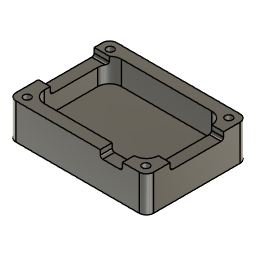
battery_holder (Autodesk Fusion 360 design; units mm, degrees)
Autodesk Fusion 360 part; units mm, degrees
sketch "Sketch1" plane through (0, 0, 0) normal (0, 0, 1) x (1, 0, 0)
  line L0 (-29, 21.25) -> (29, 21.25)
  line L1 (29, 21.25) -> (29, -21.25)
  line L2 (29, -21.25) -> (-29, -21.25)
  line L3 (-29, -21.25) -> (-29, 21.25)
  line L4 (24, -16.25) -> (-24, -16.25)
  line L5 (-24, -16.25) -> (-24, 16.25)
  line L6 (-24, 16.25) -> (24, 16.25)
  line L7 (24, 16.25) -> (24, -16.25)
  dimension "d1" = 58
  dimension "d2" = 42.5
  dimension "d3" = 21.25
  dimension "d4" = 29
  dimension "d5" = 5
  constraint horizontal L0
  constraint vertical L1
  constraint horizontal L2
  constraint vertical L3
  measures "d1" distance of L0.start L0.end
  measures "d2" distance of L0.start L2.end
  measures "d3" distance of origin L0
  measures "d4" distance of origin L3
extrude "Extrude1" add sketch "Sketch1" along normal blind 10
sketch "Sketch2" plane through (0, 0, 10) normal (0, 0, 1) x (-1, 0, 0)
  line L0 (24, -16.25) -> (-24, -16.25)
  line L1 (-24, -16.25) -> (-24, 16.25)
  line L2 (-24, 16.25) -> (24, 16.25)
  line L3 (24, 16.25) -> (24, -16.25)
  line L4 (29, 21.25) -> (-29, 21.25)
  line L5 (-29, 21.25) -> (-29, -21.25)
  line L6 (-29, -21.25) -> (29, -21.25)
  line L7 (29, -21.25) -> (29, 21.25)
  circle A0 centre (25, 17.5) radius 1.525
  line L8 (0, -2.5) -> (0, -20)
  circle A1 centre (-25, 17.5) radius 1.525
  line L9 (-20, 0) -> (-2.5, 0)
  circle A2 centre (-25, -17.5) radius 1.525
  circle A3 centre (25, -17.5) radius 1.525
  dimension "d8" = 3.05
  dimension "d9" = 4
  dimension "d10" = 3.75
  constraint symmetric A0 L8 A1
  constraint symmetric A0 L9 A3
  constraint symmetric A1 L9 A2
  measures "d8" diameter of A0
  measures "d9" distance of L7 A0.centre
  measures "d10" distance of L4 A0.centre
fillet "Fillet1" radius 5 4 edges at (-24, -16.25, 5) (-24, 16.25, 5) (24, 16.25, 5) (24, -16.25, 5)
extrude "Extrude2" cut sketch "Sketch2" against normal blind 19 contours A0 | A1 | A2 | A3
sketch "Sketch3" plane through (0, 0, 10) normal (0, 0, 1) x (-1, 0, 0)
  circle A0 centre (25, -17.5) radius 1.525
  circle A1 centre (-25, 17.5) radius 1.525
  circle A2 centre (25, 17.5) radius 1.525
  circle A3 centre (-25, -17.5) radius 1.525
  line L0 (19, -16.25) -> (-19, -16.25)
  arc A4 (-24, -11.25) -> (-19, -16.25) centre (-19, -11.25) ccw
  line L1 (-24, -11.25) -> (-24, 11.25)
  arc A5 (-19, 16.25) -> (-24, 11.25) centre (-19, 11.25) ccw
  line L2 (-19, 16.25) -> (19, 16.25)
  arc A6 (24, 11.25) -> (19, 16.25) centre (19, 11.25) ccw
  line L3 (24, 11.25) -> (24, -11.25)
  arc A7 (19, -16.25) -> (24, -11.25) centre (19, -11.25) ccw
  line L4 (29, 21.25) -> (-29, 21.25)
  line L5 (-29, 21.25) -> (-29, -21.25)
  line L6 (-29, -21.25) -> (29, -21.25)
  line L7 (29, -21.25) -> (29, 21.25)
  line L8 (24, 8.75) -> (29, 8.75)
  line L9 (29, 8.75) -> (29, -14.75)
  line L10 (29, -14.75) -> (24, -14.75)
  line L11 (24, -14.75) -> (24, 8.75)
  dimension "d15" = 6.5
  dimension "d16" = 12.5
  constraint horizontal L8
  constraint vertical L9
  constraint horizontal L10
  constraint vertical L11
  constraint coincident L7 L9.end
  constraint coincident L3 L8.start
  measures "d15" distance of L6 L10
  measures "d16" distance of L4 L8
extrude "Extrude3" cut sketch "Sketch3" against normal blind 3 contours L3 L7 L8 L9 L10 L11
sketch "Sketch4" plane through (0, 0, 10) normal (0, 0, 1) x (-1, 0, 0)
  line L0 (29, -14.75) -> (24, -14.75)
  arc A0 (19, -16.25) -> (24, -11.25) centre (19, -11.25) ccw
  line L1 (19, -16.25) -> (-19, -16.25)
  arc A1 (-24, -11.25) -> (-19, -16.25) centre (-19, -11.25) ccw
  line L2 (-24, -11.25) -> (-24, 11.25)
  arc A2 (-19, 16.25) -> (-24, 11.25) centre (-19, 11.25) ccw
  line L3 (-19, 16.25) -> (19, 16.25)
  arc A3 (24, 11.25) -> (19, 16.25) centre (19, 11.25) ccw
  line L4 (24, 11.25) -> (24, 8.75)
  line L5 (24, 8.75) -> (29, 8.75)
  line L6 (29, 8.75) -> (29, 21.25)
  line L7 (29, 21.25) -> (-29, 21.25)
  line L8 (-29, 21.25) -> (-29, -21.25)
  line L9 (-29, -21.25) -> (29, -21.25)
  line L10 (29, -21.25) -> (29, -14.75)
  circle A4 centre (-25, -17.5) radius 1.525
  circle A5 centre (25, 17.5) radius 1.525
  circle A6 centre (-25, 17.5) radius 1.525
  circle A7 centre (25, -17.5) radius 1.525
  line L11 (-24, 11.25) -> (-29, 11.25)
  line L12 (-29, 11.25) -> (-29, -11.25)
  line L13 (-29, -11.25) -> (-24, -11.25)
  line L14 (-24, -11.25) -> (-24, 11.25)
  line L15 (24, -14.75) -> (24, -11.25)
  dimension "d19" = 22.5
  constraint horizontal L11
  constraint vertical L12
  constraint horizontal L13
  constraint vertical L14
  constraint coincident L8 L12.end
  constraint coincident L2.end A2.end
  measures "d19" distance of L11.end L12.end
extrude "Extrude4" cut sketch "Sketch4" against normal blind 3 contours L2 L8 L11 L12 L13 L14
sketch "Sketch6" plane through (0, 0, 10) normal (0, 0, 1) x (-1, 0, 0)
  line L0 (-29, 11.25) -> (-24, 11.25)
  arc A0 (-19, 16.25) -> (-24, 11.25) centre (-19, 11.25) ccw
  line L1 (-19, 16.25) -> (19, 16.25)
  arc A1 (24, 11.25) -> (19, 16.25) centre (19, 11.25) ccw
  line L2 (24, 11.25) -> (24, 8.75)
  line L3 (24, 8.75) -> (29, 8.75)
  line L4 (29, 8.75) -> (29, 21.25)
  line L5 (29, 21.25) -> (-29, 21.25)
  line L6 (-29, 21.25) -> (-29, 11.25)
  circle A2 centre (25, 17.5) radius 1.525
  circle A3 centre (-25, 17.5) radius 1.525
  line L7 (-9.57, 16.25) -> (-18.9, 16.25)
  line L8 (-18.9, 16.25) -> (-18.9, 21.25)
  line L9 (-18.9, 21.25) -> (-9.57, 21.25)
  line L10 (-9.57, 21.25) -> (-9.57, 16.25)
  dimension "d22" = 10.1
  dimension "d23" = 9.33
  constraint horizontal L7
  constraint vertical L8
  constraint horizontal L9
  constraint vertical L10
  constraint coincident L5 L8.end
  constraint coincident L1 L7.start
  measures "d22" distance of L6 L8
  measures "d23" distance of L8.end L9.end
extrude "Extrude5" cut sketch "Sketch6" against normal blind 3 contours L1 L5 L7 L8 L9 L10
fillet "Fillet2" radius 1 6 edges at (9.57, -18.75, 7) (18.9, -18.75, 7) (-26.5, -8.75, 7) (-26.5, 14.75, 7) (26.5, 11.25, 7) (26.5, -11.25, 7)
extrude "Extrude6" cut 1 faces at (-24, 12.0833, 8) along direction (1, 0, 0) blind 4.5
fillet "Fillet3" radius 3 4 edges at (-29, 21.25, 5) (-29, -21.25, 5) (29, -21.25, 5) (29, 21.25, 5)
sketch "Sketch8" plane through (0, 0, 0) normal (0, 0, -1) x (1, 0, 0)
  arc A0 (26, -21.25) -> (29, -18.25) centre (26, -18.25) ccw
  line L0 (29, -18.25) -> (29, 18.25)
  arc A1 (29, 18.25) -> (26, 21.25) centre (26, 18.25) ccw
  line L1 (26, 21.25) -> (-26, 21.25)
  arc A2 (-26, 21.25) -> (-29, 18.25) centre (-26, 18.25) ccw
  line L2 (-29, 18.25) -> (-29, -18.25)
  arc A3 (-29, -18.25) -> (-26, -21.25) centre (-26, -18.25) ccw
  line L3 (-26, -21.25) -> (26, -21.25)
  circle A4 centre (-25, -17.5) radius 1.525
  circle A5 centre (25, 17.5) radius 1.525
  circle A6 centre (-25, 17.5) radius 1.525
  circle A7 centre (25, -17.5) radius 1.525
  arc A8 (-24, -11.25) -> (-19, -16.25) centre (-19, -11.25) ccw
  line L4 (-24, -11.25) -> (-24, 11.25)
  arc A9 (-19, 16.25) -> (-24, 11.25) centre (-19, 11.25) ccw
  line L5 (-19, 16.25) -> (19, 16.25)
  arc A10 (24, 11.25) -> (19, 16.25) centre (19, 11.25) ccw
  line L6 (24, 11.25) -> (24, -11.25)
  arc A11 (19, -16.25) -> (24, -11.25) centre (19, -11.25) ccw
  line L7 (19, -16.25) -> (-19, -16.25)
  line L8 (-29, 21.25) -> (29, 21.25)
  line L9 (29, 21.25) -> (29, -21.25)
  line L10 (29, -21.25) -> (-29, -21.25)
  line L11 (-29, -21.25) -> (-29, 21.25)
  dimension "d32" = 42.5
  dimension "d33" = 21.25
  constraint horizontal L8
  constraint vertical L9
  constraint horizontal L10
  constraint vertical L11
  constraint coincident L0 L9.end
  constraint coincident L2 L8.start
  measures "d32" distance of L8.start L10.end
  measures "d33" distance of origin L8
extrude "Extrude7" add sketch "Sketch8" 1 faces at (-6.3333, -19.5833, 0) along normal blind 5 contours A8 L4 A9 L5 A10 L6 A11 L7
sketch "Sketch9" plane through (0, 0, -5) normal (0, 0, -1) x (1, 0, 0)
  arc A0 (26, -21.25) -> (29, -18.25) centre (26, -18.25) ccw
  line L0 (29, -18.25) -> (29, 18.25)
  arc A1 (29, 18.25) -> (26, 21.25) centre (26, 18.25) ccw
  line L1 (26, 21.25) -> (-26, 21.25)
  arc A2 (-26, 21.25) -> (-29, 18.25) centre (-26, 18.25) ccw
  line L2 (-29, 18.25) -> (-29, -18.25)
  arc A3 (-29, -18.25) -> (-26, -21.25) centre (-26, -18.25) ccw
  line L3 (-26, -21.25) -> (26, -21.25)
  circle A4 centre (-25, -17.5) radius 1.525
  circle A5 centre (25, 17.5) radius 1.525
  circle A6 centre (-25, 17.5) radius 1.525
  circle A7 centre (25, -17.5) radius 1.525
  circle A8 centre (-25, 17.5) radius 2.85
  circle A9 centre (-25, -17.5) radius 2.85
  circle A10 centre (25, 17.5) radius 2.85
  circle A11 centre (25, -17.5) radius 2.75
  dimension "d36" = 5.7
  dimension "d37" = 5.7
  dimension "d38" = 5.7
  dimension "d39" = 5.5
  constraint concentric A6 A8
  constraint concentric A4 A9
  constraint concentric A5 A10
  constraint concentric A7 A11
  measures "d36" diameter of A8
  measures "d37" diameter of A9
  measures "d38" diameter of A10
  measures "d39" diameter of A11
extrude "Extrude8" cut sketch "Sketch9" against normal blind 6 contours A8 | A9 | A10 | A11
equation "d3 = ( 42.5 / 2 ) * 1 mm"
equation "d33 = ( 42.5 / 2 ) * 1 mm"
